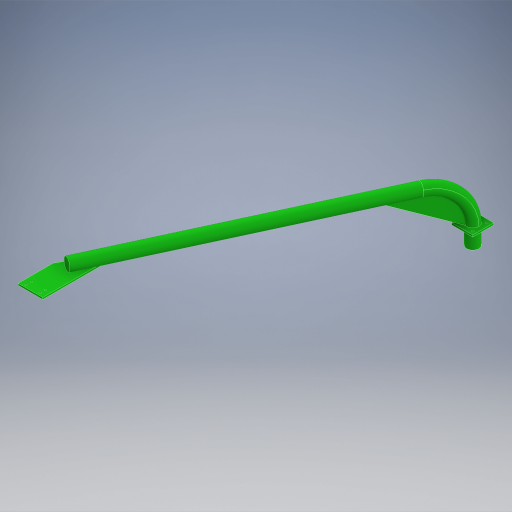
# Autodesk Inventor part: Soporte Lateral
Saved by Autodesk Inventor 2024.3 (Build 283343010, 343A)
## iProperties
Created: 2025-05-04
Part Number: Soporte Lateral
Material: Steel, Mild
Document SubType Name: Modeling
Designer: Gary
Density: 7.85 g/cm^3
Appearance: Dark Green
Author: Gary
Autodesk Inventor part; units mm, degrees
sketch "Sketch2" plane through (0, 0, 0) normal (0, 1, 0) x (-1, 0, 0)
  line L0 (60, 60) -> (-60, 60)
  line L1 (-60, 60) -> (-60, -60)
  line L2 (-60, -60) -> (60, -60)
  line L3 (60, -60) -> (60, 60)
  line L4 (60, 60) -> (-60, -60) construction
  line L5 (-60, 60) -> (60, -60) construction
  point P0 (0, 0)
  dimension "d0" = 120
  dimension "d1" = 120
  constraints: 12 end point, 2 midpoint, 2 parallel, 1 horizontal, 1 perpendicular
  measures "d0" distance of L2.end L1.end
  measures "d1" distance of L1.end L0.end
extrude "Extrusion1" add sketch "Sketch2" along normal blind 10
sketch "Sketch3" plane through (0, 10, 0) normal (0, 1, 0) x (1, 0, 0)
  circle A0 centre (0, 0) radius 35
  dimension "d4" = 70
  constraints: 1 centre point, 1 coincident
  measures "d4" diameter of A0
extrude "Extrusion2" add sketch "Sketch3" along normal blind 0.1
ref_plane "Work Plane1" through (0, 233, 0) normal (0, 1, 0) x (1, 0, 0)
sketch "Sketch6" plane through (0, 233, 0) normal (0, 1, 0) x (1, 0, 0)
  circle A0 centre (0, 0) radius 35 projected
  line L0 (-761.7868, -1569.3508) -> (-125.1232, -187.8781)
  line L1 (-93.3364, -202.5273) -> (-125.1232, -187.8781)
  line L2 (-730, -1584) -> (-93.3364, -202.5273)
  line L3 (-730, -1584) -> (-761.7868, -1569.3508)
  constraints: 8 end point, 1 parallel, 1 perpendicular
revolve "Revolution1" add sketch "Sketch6" angle 360 about axis through (-730, 233, 1584) along (0.4185491, 0, -0.9081942) contours L0 L1 L2 L3
ref_plane "Work Plane2" through (-60, 10, 0) normal (0, 0, -1) x (0, 1, 0)
ref_plane "Work Plane3" through (0, 10.1, 0) normal (-0.9081942, 0, -0.4185491) x (0, 1, 0)
sketch "Sketch10" plane through (0, 10.1, 0) normal (-0.9081942, 0, -0.4185491) x (0, 1, 0)
  line L0 (257.9, -223) -> (187.9, -223) projected
  line L1 (-0.1, -29.3787) -> (-0.1, 79.6046) projected
  arc A0 (222.9, -223) -> (-0.1, 0) centre (-0.1, -223) ccw
  point P0 (-10.1, 0)
  dimension "d20" = 223
  dimension "d21" = 223
  constraints: 2 point on circle, 1 centre point, 1 midpoint, 1 point on line
  measures "d20" radius of A0
  measures "d21" distance from line of A0.end L0
sketch "Sketch11" plane through (0, 10.1, 0) normal (0, 1, 0) x (1, 0, 0)
  circle A0 centre (0, 0) radius 35
  constraints: 1 centre point, 1 coincident
sweep "Sweep1" add profiles "Sketch11" path "Sketch10" path curves A0
ref_plane "Work Plane4" through (0, 198, 0) normal (0, 1, 0) x (1, 0, 0)
sketch "Sketch13" plane through (0, 198, 0) normal (0, 1, 0) x (1, 0, 0)
  line L0 (0, 0) -> (-730, -1584)
  line L1 (-761.7868, -1569.3508) -> (-125.1232, -187.8781) projected
  line L2 (-740, -1683.1667) -> (-740, -1753.7056)
  line L3 (-730, -1584) -> (-670, -1584)
  line L4 (-670, -1584) -> (-670, -1782.3333)
  line L5 (-670, -1782.3333) -> (-810, -1782.3333)
  line L6 (-810, -1782.3333) -> (-810, -1584)
  line L7 (-810, -1584) -> (-670, -1782.3333) construction
  line L8 (-670, -1584) -> (-810, -1782.3333) construction
  line L9 (-670, -1584) -> (-790, -1584)
  line L10 (-731.545, -1444) -> (-670, -1444)
  line L11 (-670, -1444) -> (-670, -1584)
  line L12 (-810, -1584) -> (-731.545, -1444)
  point P0 (-670, -1453.8082)
  dimension "d25" = 170
  dimension "d26" = 140
  dimension "d29" = 10.475
  dimension "d32" = 140
  dimension "d33" = 670
  dimension "d34" = 1444
  dimension "d44" = 175.477
  dimension "d45" = 19.4916
  constraints: 24 end point, 5 parallel, 3 midpoint, 2 horizontal, 1 perpendicular, 1 vertical
  measures "d25" distance of L0.end L2.end
  measures "d26" distance of L4.end L5.end
  measures "d29" angle of L8 L1
  measures "d32" distance between parallel lines of L10 L3
  measures "d33" distance from line of L0.start L4
  measures "d34" distance from line of L0.start L10
  measures "d44" angle of L12 L1
  measures "d45" distance from line of L9.end L1
extrude "Extrusion3" add sketch "Sketch13" against normal blind 10
sketch "Sketch14" plane through (0, 10.1, 0) normal (-0.9081942, 0, -0.4185491) x (0, 1, 0)
  line L0 (0, -35) -> (0, 35) projected
  line L1 (0, -35) -> (187.9, -388.1196)
  line L2 (187.9, -1744.1204) -> (187.9, -223) projected
  line L3 (187.9, -388.1196) -> (187.9, -77.6275)
  arc A0 (237.5492, -222.9934) -> (0, 14.6492) centre (-0.1, -223) ccw projected
  line L4 (112.9166, -13.9441) -> (0, -35)
  line L5 (112.9166, -13.9441) -> (187.9, -77.6275)
  point P0 (-10.1, 0)
  point P1 (187.9, -223)
  dimension "d37" = 151.982
  dimension "d38" = 79.437
  constraints: 8 end point, 2 point on circle, 1 point on line, 1 vertical
  measures "d37" angle of L0 L1
  measures "d38" angle of L4 L2
extrude "Extrusion4" add sketch "Sketch14" along normal mid plane 10 separate body contours L4 L5 L3 L2 L1
sketch "Sketch15" plane through (0, 188, 0) normal (0, -1, 0) x (1, 0, 0)
  circle A0 centre (-700, 1737.3333) radius 5.5
  circle A1 centre (-780, 1737.3333) radius 5.5
  circle A2 centre (-700, 1767.3333) radius 5.5
  circle A3 centre (-780, 1767.3333) radius 5.5
  line L0 (-670, 1444) -> (-670, 1782.3333) projected
  line L1 (-670, 1782.3333) -> (-810, 1782.3333) projected
  point P0 (0, 0)
  dimension "d46" = 30
  dimension "d47" = 15
  dimension "d48" = 11
  dimension "d49" = 11
  dimension "d50" = 11
  dimension "d51" = 11
  dimension "d52" = 80
  dimension "d53" = 30
  constraints: 4 centre point, 2 horizontal alignment, 2 vertical alignment
  measures "d46" distance from line of L0 A0.centre
  measures "d47" distance from line of L1 A3.centre
  measures "d48" diameter of A0
  measures "d49" diameter of A2
  measures "d50" diameter of A3
  measures "d51" diameter of A1
  measures "d52" distance of A1.centre A0.centre
  measures "d53" distance of A2.centre A0.centre
extrude "Extrusion5" cut sketch "Sketch15" against normal up to next bodies 1
sketch "Sketch16" plane through (0, 0, 0) normal (0, -1, 0) x (1, 0, 0)
  circle A0 centre (40, -40) radius 5.5
  circle A1 centre (-40, -40) radius 5.5
  circle A2 centre (40, 40) radius 5.5
  circle A3 centre (-40, 40) radius 5.5
  line L0 (60, 60) -> (60, -60) projected
  line L1 (60, -60) -> (-60, -60) projected
  line L2 (-60, -60) -> (-60, 60) projected
  line L3 (-60, 60) -> (60, 60) projected
  point P0 (0, 0)
  dimension "d56" = 11
  dimension "d57" = 20
  dimension "d58" = 20
  dimension "d59" = 20
  dimension "d60" = 20
  dimension "d61" = 11
  dimension "d62" = 11
  dimension "d63" = 11
  constraints: 4 centre point, 2 horizontal alignment, 2 vertical alignment
  measures "d56" diameter of A0
  measures "d57" distance from line of L0 A0.centre
  measures "d58" distance from line of L1 A0.centre
  measures "d59" distance from line of L2 A1.centre
  measures "d60" distance from line of L3 A2.centre
  measures "d61" diameter of A2
  measures "d62" diameter of A3
  measures "d63" diameter of A1
extrude "Extrusion6" cut sketch "Sketch16" against normal blind 10 contours A0 | A1 | A2 | A3 bodies 1
sketch "Sketch17" plane through (0, 0, 0) normal (0, -1, 0) x (1, 0, 0)
  circle A0 centre (0, 0) radius 35
  dimension "d66" = 70
  constraints: 1 centre point, 1 coincident
  measures "d66" diameter of A0
extrude "Extrusion7" add sketch "Sketch17" along normal blind 100 bodies 1
body "Solid1"
body "Solid2"
